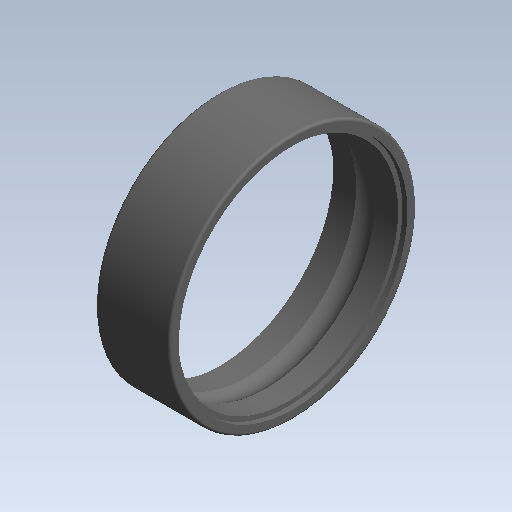
# Autodesk Inventor part: MR106ZZ1 Outer Ring
Saved by Autodesk Inventor 2021.3 (Build 253353010, 353A)
## iProperties
Part Number: MR106ZZ1 Outer Ring
Material: 一般
Catalog Web Link: www.cadenas.de
Description: shielde_type_zz_zzs_OR-
Vendor: NSK_RB
Document SubType Name: Modeling
Designer: partserver
Manufacturer: NSK_RB
Mass: 0.0445508 g
Surface Area: 2.11114 cm^2
Volume: 0.0445508 cm^3
Density: 1 g/cm^3
Appearance: PSOLRGB-128-128-128
Category: PARTsolutions
Company: NSK_RB
PSOL_IDENT_0: {$CADENAS_DATA\23d-libs\nsk_rb\roller_bearings\deep_groove_bb\exstra_small_miniatur_bb\metric_design
PSOL_IDENT_1: \shielded_type_zz_zzs_or.prj},195 {VTYP=3D},{NB=MR106ZZ1 Outer Ring},{LINA=MR106ZZ1 Outer Ring},{NN=
PSOL_IDENT_2: shielde_type_zz_zzs_OR},{DATE=25.05.2021 06:41:25},{GEOMDATE=04.01.2008 00:00:00},{VERSION=},{LINEID=
PSOL_IDENT_3: 600},{WBVAR=},{WBNUMERIC=}  {NB=MR106ZZ1 Outer Ring},{LINA=MR106ZZ1 Outer Ring},{KT=DUMMY},{IDNR=},{
PSOL_IDENT_4: STAN=Standard},{ORDER=MR106ZZ1},{SD=6.0},{X=6.0},{DI1=7.04},{DI2=7.04},{SDE1=8.90},{SDE2=9.25},{D=10
PSOL_IDENT_5: },{DD=10},{B=2.5},{B1=3.0},{R=0.15},{R1=0.10},{CR1=495},{COR1=218},{CR2=51},{COR2=22.0},{LG=45000},{
PSOL_IDENT_6: LO=53000},{DA=0.0},{DB=7.0},{DA1=0.0},{DB1=9.3},{RA=0.00},{RB=0.10},{MASS=0.68},{SC=1}
NB: MR106ZZ1 Outer Ring
NN: shielde_type_zz_zzs_OR
NBSYN: $ORDER. Outer Ring
LINA: MR106ZZ1 Outer Ring
CATALOG: NSK Rolling Bearing
STAN: Standard
ORDER: MR106ZZ1
SD: 6
X: 6
DI1: 7.04
DI2: 7.04
SDE1: 8.9
SDE2: 9.25
D: 10
DD: 10
B: 2.5
B1: 3
R: 0.15
R1: 0.1
CR1: 495
COR1: 218
CR2: 51
COR2: 22
LG: 45000
LO: 53000
DA: 0
DB: 7
DA1: 0
DB1: 9.3
RA: 0
RB: 0.1
MASS: 0.68
SC: 1
SUPPLIER: NSK_RB
ARTICLENO: MR106ZZ1 Outer Ring
BOMINFO: MR106ZZ1 Outer Ring
CREATOR: CADENAS GmbH
Title: MR106ZZ1 Outer Ring
Author: Cadenas PARTsolutions
Autodesk Inventor part; units mm, degrees
sketch "Sketch_1" plane through (0, 0, 0) normal (0, 0, 1) x (1, 0, 0)
  line L0 (3, 0) -> (0, 0)
  line L1 (0, 4.625) -> (0.1992, 4.625)
  line L2 (0.1992, 4.625) -> (0.1992, 4.45)
  line L3 (0.1992, 4.45) -> (1.1031, 4.45)
  arc A0 (1.8969, 4.45) -> (1.1031, 4.45) centre (1.5, 4) ccw
  line L4 (1.8969, 4.45) -> (2.8008, 4.45)
  line L5 (2.8008, 4.45) -> (2.8008, 4.625)
  line L6 (2.8008, 4.625) -> (3, 4.625)
  line L7 (3, 4.625) -> (3, 4.9)
  arc A1 (3, 4.9) -> (2.9, 5) centre (2.9, 4.9) ccw
  line L8 (2.9, 5) -> (0.1, 5)
  arc A2 (0.1, 5) -> (0, 4.9) centre (0.1, 4.9) ccw
  line L9 (0, 4.9) -> (0, 4.625)
  constraints: 20 end point, 6 point on circle, 3 centre point
revolve "Revolution1" add sketch "Sketch_1" angle 360 about axis through (3, 0, 0) along (1, 0, 0)
ref_plane "ip_st_or_1_XY" through (0, 0, 0) normal (1, 0, 0) x (0, 0, -1)
ref_plane "ip_st_or_1_YZ" through (0, 0, 0) normal (0, 0, -1) x (0, 1, 0)
ref_plane "ip_st_or_1_ZX" through (0, 0, 0) normal (0, 1, 0) x (1, 0, 0)
ref_plane "ip_st_or_2_XY" through (2.8008, 0, 0) normal (-1, 0, 0) x (0, 0, -1)
ref_plane "ip_st_or_2_YZ" through (2.8008, 0, 0) normal (0, 0, -1) x (0, -1, 0)
ref_plane "ip_st_or_2_ZX" through (2.8008, 0, 0) normal (0, -1, 0) x (-1, 0, 0)
body "Solid1"
